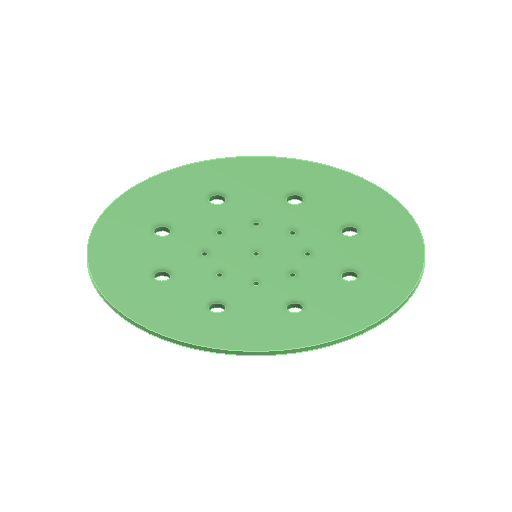
# Autodesk Inventor part: CUT_FR4_Top_Disc_PCB
Saved by Autodesk Inventor 2026.1 (Build 301233000, 233)
## iProperties
Created: 2025-06-17
Part Number: CUT_FR4_Top_Disc_PCB
Material: Generic
Document SubType Name: Modeling
Designer: User
Density: 1 g/cm^3
Appearance: Smooth - Dark Forest Green
Author: User
Autodesk Inventor part; units mm, degrees
ref_plane "XZ Plane" through (0, 0, 0) normal (0, 1, 0) x (-1, 0, 0)
ref_plane "XY Plane" through (0, 0, 0) normal (0, 0, 1) x (1, 0, 0)
sketch "Sketch1" plane through (0, 0, 0) normal (0, 1, 0) x (-1, 0, 0)
  circle A0 centre (0, 0) radius 50
  dimension "d0" = 100
  constraints: 1 centre point, 1 coincident
  measures "d0" diameter of A0
extrude "Extrusion1" add sketch "Sketch1" along normal blind 20
ref_plane "Work Plane1" through (50, 0, 0) normal (1, 0, 0) x (0, 1, 0)
sketch "Sketch2" plane through (50, 0, 0) normal (1, 0, 0) x (0, 1, 0)
  line L0 (20, -50) -> (20, 50) projected
  line L1 (0, -50) -> (0, 50) projected
  point P0 (0, 0)
  point P1 (10, 0)
  dimension "d3" = 20
  dimension "d4" = 10
  measures "d3" distance between parallel lines of L1 L0
  measures "d4" distance from line of L0 point (10, 0)
hole "Hole1" at (50, 10, 0) direction (-1, 0, 0) diameter 10 end through all
pattern_circular "Circular Pattern2" count 8 over 360 about axis through (0, -10, 0) along (0, 1, 0) of "Hole1"
sketch "Sketch4" plane through (0, 0, 0) normal (0, -1, 0) x (1, 0, 0)
  circle A0 centre (0, 0) radius 1
  dimension "d26" = 2
  constraints: 1 centre point, 1 coincident
  measures "d26" diameter of A0
extrude "Extrusion2" cut sketch "Sketch4" against normal through all
sketch "Sketch5" plane through (0, 0, 0) normal (0, -1, 0) x (1, 0, 0)
  circle A0 centre (0, 0) radius 1 projected
  line L0 (-11.4805, 27.7164) -> (0, 0)
  line L1 (0, 0) -> (0, 50)
  circle A1 centre (0, 0) radius 50 projected
  point P0 (-27.7164, 11.4805)
  point P1 (-27.7164, -11.4805)
  point P2 (-11.4805, -27.7164)
  point P3 (11.4805, -27.7164)
  point P4 (27.7164, -11.4805)
  point P5 (27.7164, 11.4805)
  point P6 (11.4805, 27.7164)
  dimension "d31" = 30
  dimension "d32" = 22.5
  dimension "d35" = 360
  constraints: 4 end point, 2 vertical, 1 vertical alignment, 10 other
  measures "d31" distance of point (0, 0) L0.start
  measures "d32" angle of L1 L0
hole "Hole3" at (-11.4805, 0, 27.7164) at (-27.7164, 0, 11.4805) at (-27.7164, 0, -11.4805) at (-11.4805, 0, -27.7164) at (11.4805, 0, -27.7164) at (27.7164, 0, -11.4805) at (27.7164, 0, 11.4805) at (11.4805, 0, 27.7164) direction (0, 1, 0) diameter 5 end through all
chamfer "Chamfer2" distance 1 angle 45 32 edges at (-49.8543, 6.7667, -3.8139) (-49.8545, 13.2353, -3.8122) (-49.8543, 13.2328, 3.8143) (-49.8544, 6.7652, 3.8126) (49.8545, 13.2353, -3.8122) (49.8543, 13.2328, 3.8143) (49.8543, 6.7667, -3.8139) (49.8544, 6.7652, 3.8126) (-37.9567, 6.7803, 32.5468) (-37.9554, 13.222, 32.5482) (-32.5468, 6.7803, 37.9567) (-32.5468, 13.2197, 37.9567) (32.5482, 13.222, -37.9554) (37.9567, 13.2197, -32.5468) (32.5468, 6.7803, -37.9567) (37.9567, 6.7803, -32.5468) (32.5468, 6.7803, 37.9567) (32.5482, 13.222, 37.9554) (37.9567, 6.7803, 32.5468) (37.9567, 13.2197, 32.5468) (-37.9554, 13.222, -32.5482) (-32.5468, 13.2197, -37.9567) (-37.9567, 6.7803, -32.5468) (-32.5468, 6.7803, -37.9567) (-3.8254, 6.7803, 49.8535) (-3.8235, 13.222, 49.8536) (3.8254, 6.7803, 49.8535) (3.8254, 13.2197, 49.8535) (-3.8235, 13.222, -49.8536) (3.8254, 13.2197, -49.8535) (-3.8254, 6.7803, -49.8535) (3.8254, 6.7803, -49.8535)
sketch "Sketch6" plane through (0, 20, 0) normal (0, 1, 0) x (1, 0, 0)
  circle A0 centre (0, 0) radius 60
  dimension "d50" = 120
  constraints: 1 centre point, 1 coincident
  measures "d50" diameter of A0
extrude "Extrusion3" cut sketch "Sketch6" against normal blind 10.25
sketch "Sketch7" plane through (0, 9.75, 0) normal (0, 1, 0) x (1, 0, 0)
  circle A0 centre (0, 0) radius 17.5
  dimension "d53" = 35
  constraints: 1 centre point, 1 coincident
  measures "d53" diameter of A0
extrude "Extrusion4" cut sketch "Sketch7" against normal blind 5
sketch "Sketch8" plane through (0, 0, 0) normal (0, -1, 0) x (1, 0, 0)
  point P0 (0, 0)
  point P1 (15.25, 0)
  point P2 (10.7834, 10.7834)
  point P3 (0, 15.25)
  point P4 (-10.7834, 10.7834)
  point P5 (-15.25, 0)
  point P6 (-10.7834, -10.7834)
  point P7 (0, -15.25)
  point P8 (10.7834, -10.7834)
  dimension "d56" = 15.25
  dimension "d59" = 360
  constraints: 9 other
  measures "d56" distance of point (15.25, 0) point (0, 0)
hole "Hole4" at (15.25, 0, 0) at (10.7834, 0, 10.7834) at (0, 0, 15.25) at (-10.7834, 0, 10.7834) at (-15.25, 0, 0) at (-10.7834, 0, -10.7834) at (0, 0, -15.25) at (10.7834, 0, -10.7834) direction (0, 1, 0) diameter 2 end through all
sketch "Sketch9" plane through (0, 9.75, 0) normal (0, 1, 0) x (1, 0, 0)
  circle A0 centre (0, 0) radius 1 projected
  circle A1 centre (0, 0) radius 60
  dimension "d68" = 120
  constraints: 1 centre point, 1 coincident
  measures "d68" diameter of A1
extrude "Extrusion5" cut sketch "Sketch9" against normal blind 8.15
equation "\"d4\" = 0.5 * d3"
body "Solid1"
